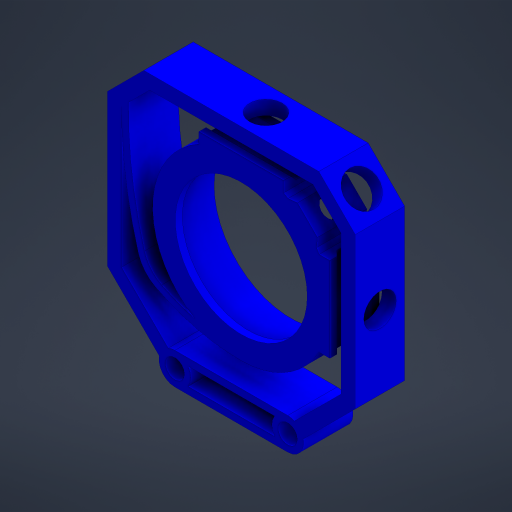
# Autodesk Inventor part: One Inch Lense Holder (V5)
Saved by Autodesk Inventor 2023.4 (Build 274418000, 418)
## iProperties
Created: 2022-07-25
Part Number: One Inch Lense Holder (V5)
Material: Generic
Document SubType Name: Modeling
Designer: xSibe
Density: 1 g/cm^3
Appearance: Plastic Blue
Author: xSibe
Autodesk Inventor part; units mm, degrees
ref_plane "YZ Plane" through (0, 0, 0) normal (1, 0, 0) x (0, 1, 0)
ref_plane "XZ Plane" through (0, 0, 0) normal (0, 1, 0) x (-1, 0, 0)
ref_plane "XY Plane" through (0, 0, 0) normal (0, 0, 1) x (1, 0, 0)
sketch "Sketch1" plane through (0, 0, 0) normal (0, 0, 1) x (1, 0, 0)
  circle A0 centre (10, 3.85) radius 1.5625 projected
  circle A1 centre (-10, 3.85) radius 1.5625 projected
  line L0 (-16.9, 0) -> (16.9, 0) projected
  line L1 (16.9, 0) -> (16.9, 7.7) projected
  line L2 (-16.9, 7.7) -> (16.9, 7.7) projected
  line L3 (-16.9, 0) -> (-16.9, 7.7) projected
  circle A2 centre (-10, 3.85) radius 2.8125
  circle A3 centre (10, 3.85) radius 2.8125
  line L4 (-10, 6.6625) -> (10, 6.6625)
  line L5 (10, 1.0375) -> (-10, 1.0375)
  line L6 (-10, 2.2875) -> (10, 2.2875)
  line L7 (-10, 5.4125) -> (10, 5.4125)
  line L8 (-17.05, 7.7) -> (-17.05, 42.1) projected
  line L9 (17.05, 7.7) -> (17.05, 42.1) projected
  line L10 (-17.05, 24.9) -> (17.05, 24.9)
  line L11 (0, 24.9) -> (1.7678, 26.6678)
  line L12 (0, 24.9) -> (2.5, 24.9) construction
  circle A4 centre (1.7678, 26.6678) radius 13.575
  circle A5 centre (1.7678, 26.6678) radius 11.075
  circle A6 centre (1.7678, 26.6678) radius 15.7
  line L13 (1.7678, 26.6678) -> (1.7678, 42.3678)
  line L14 (1.7678, 42.3678) -> (1.7678, 41.3678)
  line L15 (-5.7322, 40.3678) -> (9.2678, 40.3678)
  line L16 (9.2678, 40.3678) -> (9.2678, 42.3678)
  line L17 (9.2678, 42.3678) -> (-5.7322, 42.3678)
  line L18 (-5.7322, 42.3678) -> (-5.7322, 40.3678)
  line L19 (-5.7322, 40.3678) -> (9.2678, 42.3678) construction
  line L20 (9.2678, 40.3678) -> (-5.7322, 42.3678) construction
  line L21 (1.7678, 26.6678) -> (12.8693, 37.7693)
  line L22 (12.8693, 37.7693) -> (12.4274, 37.3274)
  line L23 (15.2558, 36.6203) -> (11.7203, 40.1558)
  line L24 (11.7203, 40.1558) -> (9.599, 38.0345)
  line L25 (9.599, 38.0345) -> (13.1345, 34.499)
  line L26 (13.1345, 34.499) -> (15.2558, 36.6203)
  line L27 (15.2558, 36.6203) -> (9.599, 38.0345) construction
  line L28 (11.7203, 40.1558) -> (13.1345, 34.499) construction
  line L29 (15.2558, 36.6203) -> (20.2558, 36.6203) construction
  line L30 (15.4678, 19.1678) -> (15.4678, 34.1678)
  line L31 (15.4678, 34.1678) -> (17.4678, 34.1678)
  line L32 (17.4678, 34.1678) -> (17.4678, 19.1678)
  line L33 (17.4678, 19.1678) -> (15.4678, 19.1678)
  line L34 (1.7678, 42.3678) -> (1.7678, 44.3678)
  line L35 (17.4678, 26.6678) -> (19.4678, 26.6678)
  line L36 (-10.2178, 5.4322) -> (10.2178, 5.4322)
  line L37 (19.4678, 14.6822) -> (19.4678, 39.3678)
  line L38 (14.4678, 44.3678) -> (-14.4678, 44.3678)
  line L39 (-19.4678, 39.3678) -> (-19.4678, 14.6822)
  line L40 (-19.4678, 5.4322) -> (19.4678, 44.3678) construction
  line L41 (19.4678, 5.4322) -> (-19.4678, 44.3678) construction
  line L42 (-10.2178, 5.4322) -> (-19.4678, 14.6822)
  line L43 (10.2178, 5.4322) -> (19.4678, 14.6822)
  line L44 (14.4678, 44.3678) -> (19.4678, 39.3678)
  line L45 (-14.4678, 44.3678) -> (-19.4678, 39.3678)
  line L46 (-15.5033, 46.8678) -> (-21.9678, 40.4033)
  line L47 (-21.9678, 40.4033) -> (-21.9678, 13.6467)
  line L48 (-21.9678, 13.6467) -> (-11.2533, 2.9322)
  line L49 (-11.2533, 2.9322) -> (11.2533, 2.9322)
  line L50 (11.2533, 2.9322) -> (21.9678, 13.6467)
  line L51 (21.9678, 13.6467) -> (21.9678, 40.4033)
  line L52 (21.9678, 40.4033) -> (15.5033, 46.8678)
  line L53 (15.5033, 46.8678) -> (-15.5033, 46.8678)
  circle A7 centre (-10, 3.85) radius 1.705
  circle A8 centre (10, 3.85) radius 1.707
  line L54 (1.7678, 10.9678) -> (-15.7322, 10.9678)
  arc A9 (-15.7322, 15.9678) -> (1.7678, 10.9678) centre (1.7678, 44.0928) ccw
  line L55 (-15.7322, 10.9678) -> (-15.7322, 15.9678)
  arc A10 (-19.4678, 39.3678) -> (-15.7322, 15.9678) centre (55.6907, 39.3678) ccw
  arc A11 (-18.207, 40.6285) -> (-14.6856, 16.7925) centre (55.6907, 39.3678) ccw
  arc A12 (-14.6856, 16.7925) -> (-6.4646, 13.2992) centre (1.7678, 44.0928) ccw
  arc A13 (-16.471, 18.3561) -> (-13.426, 14.6578) centre (-10.6407, 20.0537) ccw
  line L56 (-15.7322, 15.9678) -> (-16.471, 18.3561)
  line L57 (-14.6856, 16.7925) -> (-15.4088, 19.1856)
  arc A14 (-15.4088, 19.1856) -> (-12.3556, 15.5175) centre (-9.7485, 20.7924) ccw
  point P0 (0, 0)
  point P1 (-18.1922, 40.6434)
  point P2 (-7.6615, 2.2875)
  point P3 (-7.6615, 5.4125)
  point P4 (7.6615, 5.4125)
  point P5 (7.6615, 2.2875)
  point P6 (7.3415, 2.9322)
  point P7 (-7.3415, 2.9322)
  point P8 (-11.1858, 6.4003)
  point P9 (11.1858, 6.4003)
  point P10 (-5.7322, 40.4605)
  point P11 (15.5605, 19.1678)
  point P12 (15.5605, 34.1678)
  point P13 (14.4955, 35.8599)
  point P14 (10.9599, 39.3955)
  point P15 (9.2678, 40.4605)
  point P16 (12.7519, 4.4308)
  point P17 (-12.7519, 4.4308)
  point P18 (-7.8312, 14.244)
  point P19 (7.6748, 5.4322)
  point P20 (-7.6748, 5.4322)
  point P21 (-16.4113, 18.1632)
  point P22 (-15.3512, 18.9951)
  point P23 (-17.05, 20.4578)
  point P24 (-17.05, 26.2814)
  point P25 (-16.7879, 24.9)
  point P26 (-17.05, 12.2645)
  point P27 (-17.05, 41.7855)
  dimension "d0" = 1.25
  dimension "d1" = 1.25
  dimension "d2" = 2.5
  dimension "d3" = 45
  dimension "d4" = 27.15
  dimension "d5" = 2.5
  dimension "d6" = 2.125
  dimension "d7" = 1
  dimension "d8" = 15
  dimension "d9" = 2
  dimension "d10" = 0.625
  dimension "d11" = 5
  dimension "d12" = 135
  dimension "d13" = 3
  dimension "d14" = 2
  dimension "d15" = 2
  dimension "d16" = 38.9355
  dimension "d17" = 38.9355
  dimension "d18" = 9.25
  dimension "d19" = 9.25
  dimension "d20" = 9.25
  dimension "d21" = 9.25
  dimension "d22" = 5
  dimension "d23" = 5
  dimension "d24" = 5
  dimension "d25" = 5
  dimension "d26" = 2.5
  dimension "d46" = 0.1425
  dimension "d47" = 0.1445
  dimension "d48" = 17.5
  dimension "d49" = 5
  dimension "d50" = 1.25
  dimension "d51" = 2.5
  dimension "d52" = 2.5
  constraints: 104 end point, 28 point on circle, 14 tangent, 13 centre point, 13 point on line, 10 midpoint, 8 parallel, 7 horizontal, 6 perpendicular, 4 symmetric about line, 2 equal length, 2 vertical, 1 coincident, 8 other
  measures "d0" radial gap between concentric circles of A1 A2
  measures "d1" radial gap between concentric circles of A0 A3
  measures "d2" distance of L11.start L11.end
  measures "d3" angle of L12 L11
  measures "d4" diameter of A4
  measures "d5" radial gap between concentric circles of A4 A5
  measures "d6" radial gap between concentric circles of A4 A6
  measures "d7" distance of L13.end L14.end
  measures "d8" distance of L17.end L16.end
  measures "d9" distance of L16.end L15.end
  measures "d10" distance of L21.end L22.end
  measures "d11" distance of L23.start L23.end
  measures "d12" angle of L29 L23
  measures "d13" distance of L24.end L23.end
  measures "d14" distance of L13.end L34.end
  measures "d15" distance of L35.start L35.end
  measures "d16" distance of L40.end L41.end
  measures "d17" distance of L41.end L40.start
  measures "d18" distance of L36.start L40.start
  measures "d19" distance of L39.end L40.start
  measures "d20" distance of L36.end L41.start
  measures "d21" distance of L37.start L41.start
  measures "d22" distance of L38.start L40.end
  measures "d23" distance of L37.end L40.end
  measures "d24" distance of L38.end L41.end
  measures "d25" distance of L39.start L41.end
  measures "d26" distance between parallel lines of L38 L53
  measures "d46" radial gap between concentric circles of A1 A7
  measures "d47" radial gap between concentric circles of A0 A8
  measures "d48" distance of L54.start L54.end
  measures "d49" distance of L54.end L55.end
  measures "d50" radial gap between concentric circles of A10 A11
  measures "d51" distance of L55.end L56.end
  measures "d52" distance of L57.start L57.end
extrude "Extrusion1" add sketch "Sketch1" along normal mid plane 8.75 contours A8 L49 A3 L7 | L7 A3 L36 A8 | A8 L43 A3 L50 | L50 A3 L6 A8 | A8 L6 A3 L49 | L7 A2 L36 A3 | L36 A3 L43 A8 | A3 L43 L2 L50 | L36 A2 L4 A3 | L7 A7 L36 A2 | A2 L49 A7 L7 | A3 L5 A2 L6 | L2 L43 L9 L50 | A2 L6 A7 L49 | L36 A7 L42 A2 | A2 L48 A7 L6 | L9 L43 L37 L44 L38 L45 L39 L42 L8 L48 L47 L46 L53 L52 L51 L50 | L42 A2 L48 L2 | L2 L48 L8 L42 | L42 A7 L48 A2 | L33 A6 L9 | L9 A6 L32 L33 | A10 L45 A11 L8 | L8 L10 A11 A12 A6 A9 A13 A10 | A6 L33 L30 L10 L9 | L9 A6 | A6 L10 A4 L30 L33 | L8 A11 L10 | L10 L30 L31 A6 L9 | A6 L9 L31 L32 | A14 A12 L57 | A6 L31 L9 | L10 A4 L25 L26 A6 L31 L30 | A6 L18 L15 L13 A4 L10 | L57 A11 | L18 L17 A6 | A6 L13 L15 L18 | L26 L25 L21 A6 | A6 L24 L23 L26 | L13 L15 L16 A6 L24 L25 A4 | L17 L16 A6 | A6 L16 L15 L13 | L21 L25 L24 A6
sketch "Sketch2" plane through (0, 0, 0) normal (0, 0, 1) x (1, 0, 0)
  circle A0 centre (1.7678, 26.6678) radius 13.575 projected
  circle A1 centre (1.7678, 26.6678) radius 11.7
  point P0 (0, 0)
  dimension "d30" = 1.875
  constraints: 1 centre point
  measures "d30" radial gap between concentric circles of A0 A1
extrude "Extrusion2" add sketch "Sketch2" against normal blind 1.25 from surface at 4.375
sketch "Sketch3" plane through (21.9678, 13.6467, -4.375) normal (1, 0, 0) x (0, 0, -1)
  line L0 (0, 5.5211) -> (-8.75, 5.5211) projected
  line L1 (0, 20.5211) -> (0, 5.5211) projected
  line L2 (0, 20.5211) -> (-8.75, 20.5211) projected
  line L3 (-8.75, 5.5211) -> (-8.75, 20.5211) projected
  line L4 (-4.375, 20.5211) -> (-4.375, 5.5211)
  circle A0 centre (-4.375, 13.0211) radius 2.875
  point P0 (-4.375, -13.6467)
  dimension "d33" = 5.75
  constraints: 3 midpoint, 2 end point, 1 centre point
  measures "d33" diameter of A0
extrude "Extrusion3" cut sketch "Sketch3" against normal up to surface (2.5 mm away) contours A0 L4 | L4 A0
sketch "Sketch4" plane through (15.5605, 34.1678, -4.375) normal (0, 1, 0) x (1, 0, 0)
  line L0 (1.9072, 0) -> (1.9072, -8.75) projected
  line L1 (0, 0) -> (1.9072, 0) projected
  line L2 (0, 0) -> (0, -8.75) projected
  line L3 (1.9072, -8.75) -> (0, -8.75) projected
  line L4 (1.9072, -8.75) -> (0, -8.75)
  line L5 (0, -8.75) -> (0, -7.5)
  line L6 (0, -7.5) -> (1.9072, -7.5)
  line L7 (1.9072, -7.5) -> (1.9072, -8.75)
  line L8 (1.9072, -7.5) -> (0, -5.5928)
  line L9 (1.9072, -7.5) -> (4.6045, -7.5) construction
  line L10 (0, -4.375) -> (1.9072, -4.375)
  line L11 (1.9072, -1.25) -> (0, -3.1572)
  line L12 (0.9536, -8.75) -> (0.9536, 0)
  point P0 (-15.5605, -4.375)
  point P1 (1.9072, -1.25)
  point P2 (0, -3.1572)
  point P3 (1.9072, -7.5)
  point P4 (0.9536, -2.2036)
  point P5 (0.9536, -6.5464)
  dimension "d36" = 1.25
  dimension "d37" = 135
  constraints: 18 end point, 4 midpoint, 2 horizontal, 2 parallel, 2 point on line, 2 symmetric about line, 1 equal length, 1 perpendicular
  measures "d36" distance of L4.end L5.end
  measures "d37" angle of L9 L8
extrude "Extrusion4" cut sketch "Sketch4" against normal up to surface (15 mm away) contours L0 L10 L12 L11 | L0 L8 L12 L10
ref_plane "Work Plane1" through (17.4678, 42.3678, 4.375) normal (0.7071068, -0.7071068, 0) x (0, 0, -1)
mirror "Mirror1" about plane through (17.4678, 42.3678, 4.375) normal (0.7071068, -0.7071068, 0) of "Extrusion3", "Extrusion4"
sketch "Sketch5" plane through (21.9678, 40.4033, 4.375) normal (0.7071068, 0.7071068, 0) x (0.7071068, -0.7071068, 0)
  line L0 (0, 8.75) -> (0, 0) projected
  line L1 (-9.1421, 8.75) -> (0, 8.75) projected
  line L2 (-9.1421, 8.75) -> (-9.1421, 0) projected
  line L3 (0, 0) -> (-9.1421, 0) projected
  line L4 (-2.0711, 8.75) -> (-2.0711, 0) projected
  line L5 (-7.0711, 8.75) -> (-2.0711, 8.75) projected
  line L6 (-7.0711, 8.75) -> (-7.0711, 0) projected
  line L7 (-2.0711, 0) -> (-7.0711, 0) projected
  circle A0 centre (-4.5711, 4.375) radius 1.875
  line L8 (-7.0711, 4.375) -> (-2.0711, 4.375)
  circle A1 centre (-4.5711, 4.375) radius 3
  point P0 (13.0359, 4.375)
  dimension "d40" = 3.75
  dimension "d41" = 6
  constraints: 3 midpoint, 2 centre point, 2 end point, 1 coincident
  measures "d40" diameter of A0
  measures "d41" diameter of A1
extrude "Extrusion5" cut sketch "Sketch5" against normal up to surface (2.5 mm away) contours A1 L4 | L4 L8 A0 L6 A1 | A1 L6 L8 A0 L4 | L6 A1 | L8 A0 | A0 L8
extrude "Extrusion6" cut sketch "Sketch5" against normal up to surface from surface at -7.421 contours L8 A0 | A0 L8 round surface about axis through (1.7678, 26.6678, 0) along (0, 0, 1) radius 13.575 far side no
chamfer "Chamfer1" distance 1.075 angle 45 2 edges at (14.4955, 35.8599, 0) (10.9599, 39.3955, 0)
equation "\"d19\" = d18"
equation "\"d20\" = d18"
equation "\"d21\" = d20"
equation "\"d23\" = d22"
equation "\"d24\" = d22"
equation "\"d25\" = d24"
body "Solid1"
